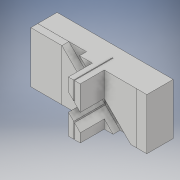
# Autodesk Inventor part: BalsaBoi2
Saved by Autodesk Inventor 2018 (Build 220112000, 112)
## iProperties
Created: 2018-08-28
Part Number: BalsaBoi2
Material: Generic
Document SubType Name: Modeling
Designer: F8PLTW
Density: 1 g/cm^3
Appearance: Default
Author: F8PLTW
Autodesk Inventor part; units mm, degrees
ref_plane "YZ Plane" through (0, 0, 0) normal (1, 0, 0) x (0, 1, 0)
ref_plane "XZ Plane" through (0, 0, 0) normal (0, 1, 0) x (-1, 0, 0)
ref_plane "XY Plane" through (0, 0, 0) normal (0, 0, 1) x (1, 0, 0)
sketch "Sketch1" plane through (0, 0, 0) normal (0, 0, 1) x (1, 0, 0)
  line L0 (-17.386, 3.6293) -> (12.614, 3.6293)
  line L1 (12.614, 3.6293) -> (12.614, -9.6107)
  line L2 (12.614, -9.6107) -> (-17.386, -9.6107)
  line L3 (-17.386, -9.6107) -> (-17.386, 3.6293)
  point P0 (0, 0)
  dimension "d0" = 30
  dimension "d1" = 13.24
  constraints: 8 end point, 2 parallel, 1 horizontal, 1 perpendicular
  measures "d0" distance of L1.end L2.end
  measures "d1" distance of L0.end L1.end
extrude "Extrusion1" add sketch "Sketch1" along normal blind 5
sketch "Sketch5" plane through (0, 0, 5) normal (0, 0, 1) x (1, 0, 0)
  line L0 (-9.3427, 3.6227) -> (3.8907, -9.6107)
  line L1 (-4.7873, 3.6293) -> (8.4461, -9.6041)
  line L2 (-4.7873, 3.6293) -> (13.9275, 3.6293) construction
  line L3 (-9.3427, 3.6227) -> (-9.3427, -9.6107)
  line L4 (-9.3427, -9.6107) -> (3.8907, -9.6107)
  line L5 (3.8907, -9.6107) -> (3.8907, -9.6107)
  line L6 (-4.7873, 3.6293) -> (9.938, 3.6293)
  line L7 (12.614, 3.6293) -> (-17.386, 3.6293) projected
  line L8 (9.938, 3.6293) -> (9.938, -9.6107)
  line L9 (-17.386, -9.6107) -> (12.614, -9.6107) projected
  line L10 (8.4461, -9.6041) -> (9.938, -9.6107)
  line L11 (-9.3427, 3.6227) -> (-9.3427, -9.6107)
  line L12 (3.8907, -9.6107) -> (-9.3427, -9.6107)
  line L13 (3.8907, -9.6107) -> (-9.3427, 3.6227)
  line L14 (-4.7873, 3.6293) -> (8.4461, -9.6041)
  line L15 (8.4461, -9.6041) -> (9.938, -9.6107)
  line L16 (9.938, 3.6293) -> (9.938, -9.6107)
  line L17 (9.938, 3.6293) -> (-4.7873, 3.6293)
  point P0 (0, 0)
  dimension "d15" = 45
  dimension "d16" = 3.2258
  dimension "d17" = 13.2334
  dimension "d18" = 18.7148
  dimension "d19" = 18.7148
  constraints: 32 end point, 8 collinear, 2 perpendicular, 2 point on line, 2 vertical, 1 equal length, 1 horizontal
  measures "d15" angle of L1 L2
  measures "d16" distance between parallel lines of L1 L0
  measures "d17" distance of L0.start L3.end
  measures "d18" distance of L0.start L0.end
  measures "d19" distance of L1.start L1.end
extrude "Extrusion5" add sketch "Sketch5" along normal blind 1.8
sketch "Sketch6" plane through (0, 0, 6.8) normal (0, 0, 1) x (1, 0, 0)
  line L0 (9.938, 3.6293) -> (-4.7873, 3.6293) projected
  line L1 (12.614, -9.6107) -> (-17.386, -9.6107) projected
  line L2 (-1.4744, 3.6293) -> (1.6007, 3.6293)
  line L3 (1.6007, 3.6293) -> (1.6007, -9.6107)
  line L4 (1.6007, -9.6107) -> (-1.4744, -9.6107)
  line L5 (-1.4744, -9.6107) -> (-1.4744, 3.6293)
  point P0 (0, 0)
  constraints: 8 end point, 2 parallel, 2 point on line, 1 horizontal, 1 perpendicular
extrude "Extrusion6" add sketch "Sketch6" along normal blind 6.2
sketch "Sketch9" plane through (0, 0, 13) normal (0, 0, 1) x (1, 0, 0)
  line L0 (-1.4744, -4.2456) -> (-9.3427, 3.6227) projected
  line L1 (-9.3427, 3.6227) -> (3.8907, -9.6107) projected
  line L2 (-1.4744, -4.2456) -> (3.8907, -9.6107)
  line L3 (3.8907, -9.6107) -> (3.8907, -5.0487)
  line L4 (8.4461, -9.6041) -> (-4.7873, 3.6293) projected
  line L5 (3.8907, -5.0487) -> (-2.9105, 1.7525)
  line L6 (-2.9105, 1.7525) -> (-2.9105, -2.8095)
  line L7 (-1.4744, -4.2456) -> (-2.9105, -2.8095)
  point P0 (0, 0)
  constraints: 10 end point, 3 point on line, 2 collinear, 1 parallel, 1 vertical
extrude "Extrusion7" cut sketch "Sketch9" against normal blind 6.3
sketch "Sketch10" plane through (0, 0, 13) normal (0, 0, 1) x (1, 0, 0)
  line L0 (12.614, -9.6107) -> (-17.386, -9.6107) projected
  line L1 (1.6007, 3.6293) -> (-1.4744, 3.6293) projected
  line L2 (-0.1, -9.6107) -> (0.1, -9.6107)
  line L3 (0.1, -9.6107) -> (0.1, 3.6293)
  line L4 (0.1, 3.6293) -> (-0.1, 3.6293)
  line L5 (-0.1, 3.6293) -> (-0.1, -9.6107)
  line L6 (0, -6.9346) -> (0, -6.5072) construction
  point P0 (0, 0)
  dimension "d26" = 0.2
  constraints: 10 end point, 2 parallel, 2 point on line, 1 horizontal, 1 perpendicular, 1 vertical, 1 other
  measures "d26" distance of L4.end L3.end
extrude "Extrusion8" cut sketch "Sketch10" against normal blind 10
sketch "Sketch11" plane through (0, 0, 5) normal (0, 0, 1) x (1, 0, 0)
  line L0 (9.938, 3.6293) -> (1.6007, 3.6293) projected
  line L1 (9.938, -9.6107) -> (12.614, -9.6107) projected
  line L2 (9.938, 3.6293) -> (12.614, 3.6293)
  line L3 (12.614, 3.6293) -> (12.614, -9.6107)
  line L4 (12.614, -9.6107) -> (9.938, -9.6107)
  line L5 (9.938, -9.6107) -> (9.938, 3.6293)
  line L6 (-17.386, -9.6107) -> (-9.3427, -9.6107) projected
  line L7 (-9.3427, 3.6227) -> (-9.3427, -9.6107) projected
  line L8 (-17.386, -9.6107) -> (-9.3427, -9.6107)
  line L9 (-9.3427, -9.6107) -> (-9.3427, 3.6227)
  line L10 (-9.3427, 3.6227) -> (-17.386, 3.6227)
  line L11 (-17.386, 3.6227) -> (-17.386, -9.6107)
  point P0 (0, 0)
  constraints: 16 end point, 4 parallel, 2 horizontal, 2 perpendicular
extrude "Extrusion9" add sketch "Sketch11" along normal blind 1.8034
body "Solid1"
